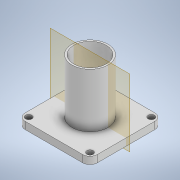
# Autodesk Inventor part: mock
Saved by Autodesk Inventor 2021 (Build 250183000, 183)
## iProperties
Created: 2022-03-11
Part Number: mock
Material: Generic
Document SubType Name: Modeling
Designer: User
Density: 1 g/cm^3
Appearance: Default
Author: User
Autodesk Inventor part; units mm, degrees
ref_plane "YZ Plane" through (0, 0, 0) normal (1, 0, 0) x (0, 1, 0)
ref_plane "XZ Plane" through (0, 0, 0) normal (0, 1, 0) x (-1, 0, 0)
sketch "Sketch1" plane through (0, 0, 0) normal (0, 1, 0) x (-1, 0, 0)
  line L0 (-8, 10) -> (8, 10)
  line L1 (10, 8) -> (10, -8)
  line L2 (8, -10) -> (-8, -10)
  line L3 (-10, -8) -> (-10, 8)
  line L4 (-10, 10) -> (10, -10) construction
  line L5 (10, 10) -> (-10, -10) construction
  arc A0 (10, 8) -> (8, 10) centre (8, 8) ccw
  arc A1 (8, -10) -> (10, -8) centre (8, -8) ccw
  arc A2 (-8, 10) -> (-10, 8) centre (-8, 8) ccw
  arc A3 (-10, -8) -> (-8, -10) centre (-8, -8) ccw
  point P0 (0, 0)
  dimension "d0" = 20
  dimension "d1" = 20
  dimension "d34" = 2
  dimension "d35" = 2
  dimension "d36" = 2
  dimension "d37" = 2
  constraints: 12 end point, 8 point on circle, 8 point on line, 8 tangent, 4 centre point, 2 midpoint, 2 parallel, 1 horizontal, 1 perpendicular
  measures "d0" distance of L4.end L5.end
  measures "d1" distance of L5.start L4.end
  measures "d34" radius of A0
  measures "d35" radius of A1
  measures "d36" radius of A2
  measures "d37" radius of A3
extrude "Extrusion1" add sketch "Sketch1" along normal blind 2
sketch "Sketch2" plane through (0, 2, 0) normal (0, 1, 0) x (1, 0, 0)
  line L0 (8.5, -8.5) -> (-8.5, -8.5)
  line L1 (-8.5, -8.5) -> (-8.5, 8.5)
  line L2 (-8.5, 8.5) -> (8.5, 8.5)
  line L3 (8.5, 8.5) -> (8.5, -8.5)
  line L4 (8.5, -8.5) -> (-8.5, 8.5) construction
  line L5 (-8.5, -8.5) -> (8.5, 8.5) construction
  point P0 (0, 0)
  dimension "d4" = 17
  dimension "d5" = 17
  constraints: 12 end point, 2 midpoint, 2 parallel, 1 horizontal, 1 perpendicular
  measures "d4" distance of L1.end L2.end
  measures "d5" distance of L0.end L1.end
hole "Hole1" at (-8.5, 2, 8.5) direction (0, -1, 0) diameter 1.778 end through all
hole "Hole2" at (8.5, 2, 8.5) direction (0, -1, 0) diameter 1.778 end through all
hole "Hole3" at (-8.5, 2, -8.5) direction (0, -1, 0) diameter 1.778 end through all
hole "Hole4" at (8.5, 2, -8.5) direction (0, -1, 0) diameter 1.778 end through all
sketch "Sketch3" plane through (0, 2, 0) normal (0, 1, 0) x (1, 0, 0)
  circle A0 centre (0, 0) radius 5
  dimension "d38" = 10
  constraints: 1 centre point, 1 coincident
  measures "d38" diameter of A0
extrude "Extrusion2" add sketch "Sketch3" along normal blind 15
sketch "Sketch4" plane through (0, 17, 0) normal (0, 1, 0) x (1, 0, 0)
  circle A0 centre (0, 0) radius 4.5
  dimension "d41" = 9
  constraints: 1 centre point, 1 coincident
  measures "d41" diameter of A0
extrude "Extrusion3" cut sketch "Sketch4" against normal blind 15
body "Solid1"
